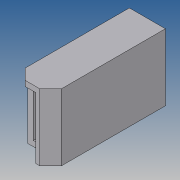
# Autodesk Inventor part: BackupBat_Wing
Saved by Autodesk Inventor 2019.4 (Build 234330000, 330)
## iProperties
Part Number: BackupBat_Wing
Material: GEDA Stahl
Document SubType Name: Modeling
Designer: Admin
Mass: 46.0856 g
Surface Area: 62.5737 cm^2
Volume: 5.8633 cm^3
Density: 7.86 g/cm^3
Appearance: GEDA Stahl A
Author: Admin
Gewicht: 0,046 kg
G_L: 0
G_H: 0
G_B: 0
InventorVersion: 2019.4
VAULT_Status: in Bearbeitung
Revision: -
Max. Breite: 0
Max. Höhe: 0
Max. Länge: 0
Max. Abmessungen: 0 x 0 x 0
Autodesk Inventor part; units mm, degrees
note: some values were not read from the file. Left out: dimensions or parameters whose unit could not be read.
ref_plane "YZ Plane" through (0, 0, 0) normal (1, 0, 0) x (0, 1, 0)
ref_plane "XZ Plane" through (0, 0, 0) normal (0, 1, 0) x (-1, 0, 0)
ref_plane "XY Plane" through (0, 0, 0) normal (0, 0, 1) x (1, 0, 0)
sketch "Skizze1" plane through (0, 0, 0) normal (0, 1, 0) x (-1, 0, 0)
  line L0 (4.75, -10.5) -> (-4.75, -10.5)
  line L1 (-4.75, -10.5) -> (-4.75, 10.5)
  line L2 (-4.75, 10.5) -> (4.75, 10.5)
  line L3 (4.75, 10.5) -> (4.75, -10.5)
  line L4 (4.75, -10.5) -> (-4.75, 10.5) construction
  line L5 (-4.75, -10.5) -> (4.75, 10.5) construction
  line L6 (-6.75, -12.5) -> (6.75, -12.5)
  line L7 (6.75, -12.5) -> (6.75, 12.5)
  line L8 (6.75, 12.5) -> (-6.75, 12.5)
  line L9 (-6.75, 12.5) -> (-6.75, -12.5)
  line L10 (-6.75, -12.5) -> (6.75, 12.5) construction
  line L11 (6.75, -12.5) -> (-6.75, 12.5) construction
  point P0 (0, 0)
  dimension "d0" = 9.5
  dimension "d1" = 21
  dimension "d2" = 2
  dimension "d3" = 2
  constraints: 24 end point, 4 midpoint, 4 parallel, 2 horizontal, 2 perpendicular
  measures "d0" distance of L1.end L2.end
  measures "d1" distance of L0.end L1.end
  measures "d2" distance between parallel lines of L3 L7
  measures "d3" distance between parallel lines of L8 L2
extrude "Extrusion1" add sketch "Skizze1" along normal blind 40
sketch "Skizze2" plane through (0, 0, 0) normal (0, -1, 0) x (1, 0, 0)
  line L0 (6.75, 12.5) -> (6.75, -12.5) projected
  line L1 (-6.75, 12.5) -> (6.75, 12.5) projected
  line L2 (-6.75, -12.5) -> (-6.75, 12.5) projected
  line L3 (-6.75, -12.5) -> (6.75, -12.5)
  line L4 (6.75, -12.5) -> (6.75, 12.5)
  line L5 (6.75, 12.5) -> (-6.75, 12.5)
  line L6 (-6.75, 12.5) -> (-6.75, -12.5)
  line L7 (-6.75, -12.5) -> (6.75, 12.5) construction
  line L8 (6.75, -12.5) -> (-6.75, 12.5) construction
  point P0 (0, 0)
  constraints: 12 end point, 2 midpoint, 2 parallel, 1 horizontal, 1 perpendicular
extrude "Extrusion2" add sketch "Skizze2" along normal blind 2
sketch "Skizze3" plane through (6.75, 40, -12.5) normal (0, 0, -1) x (-1, 0, 0)
  line L0 (11.5, -40) -> (11.5, 0) projected
  line L1 (2, -40) -> (2, 0) projected
  line L2 (11.5, -40) -> (2, -40)
  line L3 (2, -40) -> (2, -37)
  line L4 (2, -37) -> (11.5, -37)
  line L5 (11.5, -37) -> (11.5, -40)
  line L6 (13.5, -42) -> (0, -42) projected
  line L7 (11.5, -37) -> (13.5, -37)
  line L8 (13.5, -37) -> (13.5, -42)
  line L9 (13.5, -42) -> (11.5, -42)
  line L10 (11.5, -42) -> (11.5, -37)
  line L11 (11.5, -40) -> (11.5, 0) projected
  line L12 (11.5, -40) -> (5.5, -40)
  line L13 (5.5, -40) -> (5.5, -42)
  line L14 (5.5, -42) -> (11.5, -42)
  line L15 (11.5, -42) -> (11.5, -40)
  point P0 (6.75, -40)
  dimension "d8" = 3
  dimension "d9" = 6
  constraints: 24 end point, 6 parallel, 3 horizontal, 3 perpendicular, 2 point on line
  measures "d8" distance of L2.end L3.end
  measures "d9" distance between parallel lines of L10 L13
extrude "Extrusion3" cut sketch "Skizze3" against normal up to surface (23 mm away)
chamfer "Fase1" distance 3 angle 45 1 edges at (4.75, 0, -1)
chamfer "Fase2" distance 4 angle 45 1 edges at (6.75, -2, 0)
chamfer "Fase3" distance 4 angle 45 1 edges at (-6.75, -2, 11.5)
fillet "Rundung1" radius 2 2 edges at (4.75, 3, -11.5) (1.25, 0, -1)
fillet "Rundung2" radius 2 1 edges at (4.75, 3, 0)
sketch "Skizze4" plane through (0, 40, 0) normal (0, 1, 0) x (1, 0, 0)
  line L0 (2.75, 12.5) -> (6.75, 12.5) projected
  line L1 (-6.75, -12.5) -> (6.75, -12.5)
  line L2 (6.75, -12.5) -> (6.75, 12.5)
  line L3 (6.75, 12.5) -> (-6.75, 12.5)
  line L4 (-6.75, 12.5) -> (-6.75, -12.5)
  line L5 (-6.75, -12.5) -> (6.75, 12.5) construction
  line L6 (6.75, -12.5) -> (-6.75, 12.5) construction
  point P0 (0, 0)
  constraints: 12 end point, 2 midpoint, 2 parallel, 1 horizontal, 1 perpendicular
extrude "Extrusion4" add sketch "Skizze4" along normal blind 1
equation "\"G_L\" = 0"
equation "\"G_H\" = 0"
equation "\"G_B\" = 0"
